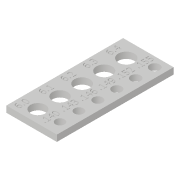
# Autodesk Inventor part: 6mm and number 6 hole test
Saved by Autodesk Inventor 2018 (Build 220112000, 112)
## iProperties
Created: 2019-07-24
Part Number: 6mm and number 6 hole test
Material: Generic
Document SubType Name: Modeling
Designer: ball
Density: 1 g/cm^3
Appearance: Default
Author: ball
Autodesk Inventor part; units mm, degrees
note: some values were not read from the file. Chosen so that the rebuilt part matches the saved one: direction of "Emboss2".
(part 1 of 2)
ref_plane "YZ Plane" through (0, 0, 0) normal (1, 0, 0) x (0, 1, 0)
ref_plane "XZ Plane" through (0, 0, 0) normal (0, 1, 0) x (-1, 0, 0)
ref_plane "XY Plane" through (0, 0, 0) normal (0, 0, 1) x (1, 0, 0)
sketch "Sketch1" plane through (0, 0, 0) normal (0, 1, 0) x (-1, 0, 0)
  line L0 (0, 0) -> (20.32, 0)
  line L1 (20.32, 0) -> (20.32, -46.99)
  line L2 (20.32, -46.99) -> (0, -46.99)
  line L3 (0, -46.99) -> (0, 0)
  circle A0 centre (3.81, -5.08) radius 1.778
  circle A1 centre (3.81, -12.7) radius 1.8161
  circle A2 centre (3.81, -20.32) radius 1.8542
  circle A3 centre (3.81, -27.94) radius 1.8923
  circle A4 centre (3.81, -35.56) radius 1.9304
  circle A5 centre (3.81, -43.18) radius 1.9685
  circle A6 centre (12.7, -5.08) radius 2.9972
  circle A7 centre (12.7, -13.97) radius 3.048
  circle A8 centre (12.7, -22.86) radius 3.0988
  circle A9 centre (12.7, -31.75) radius 3.1496
  circle A10 centre (12.7, -40.64) radius 3.2004
  dimension "d0" = 46.99
  dimension "d1" = 3.556
  dimension "d2" = 5.08
  dimension "d3" = 3.81
  dimension "d4" = 3.6322
  dimension "d5" = 12.7
  dimension "d6" = 3.7084
  dimension "d7" = 3.7846
  dimension "d8" = 3.8608
  dimension "d9" = 3.937
  dimension "d12" = 5.9944
  dimension "d13" = 20.32
  dimension "d14" = 12.7
  dimension "d15" = 5.08
  dimension "d16" = 6.096
  dimension "d17" = 6.1976
  dimension "d18" = 6.2992
  dimension "d19" = 6.4008
  dimension "d20" = 13.97
  dimension "d21" = 22.86
  dimension "d22" = 31.75
  dimension "d23" = 40.64
  dimension "d24" = 43.18
  dimension "d25" = 35.56
  dimension "d26" = 27.94
  dimension "d27" = 20.32
  constraints: 11 centre point, 8 end point, 2 parallel, 1 horizontal, 1 perpendicular
  measures "d0" distance of L0.end L1.end
  measures "d1" diameter of A0
  measures "d2" distance from line of L0 A0.centre
  measures "d3" distance from line of L3 A0.centre
  measures "d4" diameter of A1
  measures "d5" distance from line of L0 A1.centre
  measures "d6" diameter of A2
  measures "d7" diameter of A3
  measures "d8" diameter of A4
  measures "d9" diameter of A5
  measures "d12" diameter of A6
  measures "d13" distance between parallel lines of L3 L1
  measures "d14" distance from line of L3 A6.centre
  measures "d15" distance from line of L0 A6.centre
  measures "d16" diameter of A7
  measures "d17" diameter of A8
  measures "d18" diameter of A9
  measures "d19" diameter of A10
  measures "d20" distance from line of L0 A7.centre
  measures "d21" distance from line of L0 A8.centre
  measures "d22" distance from line of L0 A9.centre
  measures "d23" distance from line of L0 A10.centre
  measures "d24" distance from line of L0 A5.centre
  measures "d25" distance from line of L0 A4.centre
  measures "d26" distance from line of L0 A3.centre
  measures "d27" distance from line of L0 A2.centre
extrude "Extrusion2" add sketch "Sketch1" along normal blind 2.54
sketch "Sketch2" plane through (0, 2.54, 0) normal (0, 1, 0) x (1, 0, 0)
  line L0 (-9.0261, 9.1663) -> (-9.0261, 15.9424) construction
  line L1 (-9.0261, 15.9424) -> (-6.3791, 15.9424) construction
  line L2 (-6.3791, 15.9424) -> (-6.3791, 9.1663) construction
  line L3 (-6.3791, 9.1663) -> (-9.0261, 9.1663) construction
  line L4 (-8.8978, 1.4309) -> (-8.8978, 8.207) construction
  line L5 (-8.8978, 8.207) -> (-6.2508, 8.207) construction
  line L6 (-6.2508, 8.207) -> (-6.2508, 1.4309) construction
  line L7 (-6.2508, 1.4309) -> (-8.8978, 1.4309) construction
  line L8 (-8.9722, 16.6379) -> (-8.9722, 23.414) construction
  line L9 (-8.9722, 23.414) -> (-6.3252, 23.414) construction
  line L10 (-6.3252, 23.414) -> (-6.3252, 16.6379) construction
  line L11 (-6.3252, 16.6379) -> (-8.9722, 16.6379) construction
  line L12 (-9.0872, 24.1029) -> (-9.0872, 30.879) construction
  line L13 (-9.0872, 30.879) -> (-6.4402, 30.879) construction
  line L14 (-6.4402, 30.879) -> (-6.4402, 24.1029) construction
  line L15 (-6.4402, 24.1029) -> (-9.0872, 24.1029) construction
  line L16 (-9.0805, 31.6084) -> (-9.0805, 38.3845) construction
  line L17 (-9.0805, 38.3845) -> (-6.4335, 38.3845) construction
  line L18 (-6.4335, 38.3845) -> (-6.4335, 31.6084) construction
  line L19 (-6.4335, 31.6084) -> (-9.0805, 31.6084) construction
  line L20 (-8.9928, 39.3571) -> (-8.9928, 46.1332) construction
  line L21 (-8.9928, 46.1332) -> (-6.3458, 46.1332) construction
  line L22 (-6.3458, 46.1332) -> (-6.3458, 39.3571) construction
  line L23 (-6.3458, 39.3571) -> (-8.9928, 39.3571) construction
  line L24 (-16.5399, 1.397) -> (-19.1869, 1.397) construction
  line L25 (-19.1869, 1.397) -> (-19.1869, 8.1731) construction
  line L26 (-19.1869, 8.1731) -> (-16.5399, 8.1731) construction
  line L27 (-16.5399, 8.1731) -> (-16.5399, 1.397) construction
  line L28 (-16.5737, 11.213) -> (-19.2208, 11.213) construction
  line L29 (-19.2208, 11.213) -> (-19.2208, 17.9891) construction
  line L30 (-19.2208, 17.9891) -> (-16.5737, 17.9891) construction
  line L31 (-16.5737, 17.9891) -> (-16.5737, 11.213) construction
  line L32 (-16.7292, 20.1372) -> (-19.3762, 20.1372) construction
  line L33 (-19.3762, 20.1372) -> (-19.3762, 26.9133) construction
  line L34 (-19.3762, 26.9133) -> (-16.7292, 26.9133) construction
  line L35 (-16.7292, 26.9133) -> (-16.7292, 20.1372) construction
  line L36 (-16.8036, 29.1425) -> (-19.4506, 29.1425) construction
  line L37 (-19.4506, 29.1425) -> (-19.4506, 35.9186) construction
  line L38 (-19.4506, 35.9186) -> (-16.8036, 35.9186) construction
  line L39 (-16.8036, 35.9186) -> (-16.8036, 29.1425) construction
  line L40 (-16.7564, 38.4315) -> (-19.4034, 38.4315) construction
  line L41 (-19.4034, 38.4315) -> (-19.4034, 45.2076) construction
  line L42 (-19.4034, 45.2076) -> (-16.7564, 45.2076) construction
  line L43 (-16.7564, 45.2076) -> (-16.7564, 38.4315) construction
  spline S0 degree 2 poles (-17.4188, 3.1878) (-17.2232, 3.1878) (-16.8918, 3.0581) (-16.7807, 2.949) knots 0 0 0 1 2 2 2
  spline S1 degree 2 poles (-16.7807, 2.949) (-16.6634, 2.8358) (-16.5419, 2.5518) (-16.5419, 2.3809) knots 0 0 0 1 2 2 2
  spline S2 degree 2 poles (-16.5419, 2.3809) (-16.5419, 2.2101) (-16.6572, 1.9281) (-16.7725, 1.821) knots 0 0 0 1 2 2 2
  spline S3 degree 2 poles (-16.7725, 1.821) (-16.9104, 1.6893) (-17.3735, 1.5411) (-17.7111, 1.5411) knots 0 0 0 1 2 2 2
  spline S4 degree 2 poles (-17.7111, 1.5411) (-18.0425, 1.5411) (-18.5756, 1.677) (-18.7732, 1.819) knots 0 0 0 1 2 2 2
  spline S5 degree 2 poles (-18.7732, 1.819) (-18.9666, 1.9569) (-19.1828, 2.3933) (-19.1828, 2.6794) knots 0 0 0 1 2 2 2
  spline S6 degree 2 poles (-19.1828, 2.6794) (-19.1828, 2.7638) (-19.1663, 2.912) (-19.1478, 2.9675) knots 0 0 0 1 2 2 2
  line L44 (-19.1478, 2.9675) -> (-18.8205, 2.9675)
  line L45 (-18.8205, 2.9675) -> (-18.8205, 2.9531)
  spline S7 degree 2 poles (-18.8205, 2.9531) (-18.8452, 2.9058) (-18.8884, 2.7329) (-18.8884, 2.6341) knots 0 0 0 1 2 2 2
  spline S8 degree 2 poles (-18.8884, 2.6341) (-18.8884, 2.3171) (-18.4603, 1.9281) (-18.0404, 1.891) knots 0 0 0 1 2 2 2
  spline S9 degree 2 poles (-18.0404, 1.891) (-18.1248, 2.0125) (-18.2174, 2.2677) (-18.2174, 2.42) knots 0 0 0 1 2 2 2
  spline S10 degree 2 poles (-18.2174, 2.42) (-18.2174, 2.5682) (-18.1577, 2.7905) (-18.0672, 2.912) knots 0 0 0 1 2 2 2
  spline S11 degree 2 poles (-18.0672, 2.912) (-17.9622, 3.0519) (-17.637, 3.1878) (-17.4188, 3.1878) knots 0 0 0 1 2 2 2
  spline S12 degree 2 poles (-17.4044, 2.842) (-17.5608, 2.842) (-17.7728, 2.7597) (-17.8469, 2.6691) knots 0 0 0 1 2 2 2
  spline S13 degree 2 poles (-17.8469, 2.6691) (-17.9004, 2.6012) (-17.9354, 2.4324) (-17.9354, 2.3439) knots 0 0 0 1 2 2 2
  spline S14 degree 2 poles (-17.9354, 2.3439) (-17.9354, 2.2245) (-17.8634, 2.0001) (-17.7954, 1.891) knots 0 0 0 1 2 2 2
  spline S15 degree 2 poles (-17.7954, 1.891) (-17.7584, 1.889) (-17.6884, 1.8849) (-17.6349, 1.8849) knots 0 0 0 1 2 2 2
  spline S16 degree 2 poles (-17.6349, 1.8849) (-17.3714, 1.8849) (-17.0483, 1.9878) (-16.9639, 2.066) knots 0 0 0 1 2 2 2
  spline S17 degree 2 poles (-16.9639, 2.066) (-16.8836, 2.138) (-16.8198, 2.2945) (-16.8198, 2.383) knots 0 0 0 1 2 2 2
  spline S18 degree 2 poles (-16.8198, 2.383) (-16.8198, 2.5888) (-17.1121, 2.842) (-17.4044, 2.842) knots 0 0 0 1 2 2 2
  line L46 (-16.5954, 4.0338) -> (-16.5954, 3.6262)
  line L47 (-16.5954, 3.6262) -> (-17.0812, 3.6262)
  line L48 (-17.0812, 3.6262) -> (-17.0812, 4.0338)
  line L49 (-17.0812, 4.0338) -> (-16.5954, 4.0338)
  spline S19 degree 2 poles (-17.8654, 6.1271) (-17.1821, 6.1271) (-16.5419, 5.7299) (-16.5419, 5.3161) knots 0 0 0 1 2 2 2
  spline S20 degree 2 poles (-16.5419, 5.3161) (-16.5419, 4.8962) (-17.1944, 4.5031) (-17.8634, 4.5031) knots 0 0 0 1 2 2 2
  spline S21 degree 2 poles (-17.8634, 4.5031) (-18.5509, 4.5031) (-19.1869, 4.9003) (-19.1869, 5.3161) knots 0 0 0 1 2 2 2
  spline S22 degree 2 poles (-19.1869, 5.3161) (-19.1869, 5.734) (-18.5282, 6.1271) (-17.8654, 6.1271) knots 0 0 0 1 2 2 2
  spline S23 degree 2 poles (-17.0915, 5.6907) (-17.2171, 5.7401) (-17.604, 5.7813) (-17.8654, 5.7813) knots 0 0 0 1 2 2 2
  spline S24 degree 2 poles (-17.8654, 5.7813) (-18.1268, 5.7813) (-18.5118, 5.7401) (-18.6414, 5.6887) knots 0 0 0 1 2 2 2
  spline S25 degree 2 poles (-18.6414, 5.6887) (-18.7711, 5.6372) (-18.9049, 5.4581) (-18.9049, 5.3161) knots 0 0 0 1 2 2 2
  spline S26 degree 2 poles (-18.9049, 5.3161) (-18.9049, 5.1741) (-18.7711, 4.9909) (-18.6373, 4.9374) knots 0 0 0 1 2 2 2
  spline S27 degree 2 poles (-18.6373, 4.9374) (-18.5076, 4.8859) (-18.1124, 4.8489) (-17.8634, 4.8489) knots 0 0 0 1 2 2 2
  spline S28 degree 2 poles (-17.8634, 4.8489) (-17.5958, 4.8489) (-17.2376, 4.8818) (-17.0977, 4.9353) knots 0 0 0 1 2 2 2
  spline S29 degree 2 poles (-17.0977, 4.9353) (-16.9659, 4.9847) (-16.8239, 5.1679) (-16.8239, 5.3161) knots 0 0 0 1 2 2 2
  spline S30 degree 2 poles (-16.8239, 5.3161) (-16.8239, 5.4561) (-16.9577, 5.6393) (-17.0915, 5.6907) knots 0 0 0 1 2 2 2
  spline S31 degree 2 poles (-17.4568, 13.0038) (-17.2612, 13.0038) (-16.9298, 12.8741) (-16.8187, 12.765) knots 0 0 0 1 2 2 2
  spline S32 degree 2 poles (-16.8187, 12.765) (-16.7013, 12.6518) (-16.5799, 12.3677) (-16.5799, 12.1969) knots 0 0 0 1 2 2 2
  spline S33 degree 2 poles (-16.5799, 12.1969) (-16.5799, 12.026) (-16.6952, 11.744) (-16.8104, 11.637) knots 0 0 0 1 2 2 2
  spline S34 degree 2 poles (-16.8104, 11.637) (-16.9483, 11.5053) (-17.4115, 11.3571) (-17.749, 11.3571) knots 0 0 0 1 2 2 2
  spline S35 degree 2 poles (-17.749, 11.3571) (-18.0804, 11.3571) (-18.6136, 11.4929) (-18.8112, 11.635) knots 0 0 0 1 2 2 2
  spline S36 degree 2 poles (-18.8112, 11.635) (-19.0046, 11.7729) (-19.2208, 12.2092) (-19.2208, 12.4953) knots 0 0 0 1 2 2 2
  spline S37 degree 2 poles (-19.2208, 12.4953) (-19.2208, 12.5797) (-19.2043, 12.7279) (-19.1858, 12.7835) knots 0 0 0 1 2 2 2
  line L50 (-19.1858, 12.7835) -> (-18.8585, 12.7835)
  line L51 (-18.8585, 12.7835) -> (-18.8585, 12.7691)
  spline S38 degree 2 poles (-18.8585, 12.7691) (-18.8832, 12.7218) (-18.9264, 12.5489) (-18.9264, 12.4501) knots 0 0 0 1 2 2 2
  spline S39 degree 2 poles (-18.9264, 12.4501) (-18.9264, 12.1331) (-18.4983, 11.744) (-18.0784, 11.707) knots 0 0 0 1 2 2 2
  spline S40 degree 2 poles (-18.0784, 11.707) (-18.1628, 11.8284) (-18.2554, 12.0837) (-18.2554, 12.236) knots 0 0 0 1 2 2 2
  spline S41 degree 2 poles (-18.2554, 12.236) (-18.2554, 12.3842) (-18.1957, 12.6065) (-18.1051, 12.7279) knots 0 0 0 1 2 2 2
  spline S42 degree 2 poles (-18.1051, 12.7279) (-18.0002, 12.8679) (-17.6749, 13.0038) (-17.4568, 13.0038) knots 0 0 0 1 2 2 2
  spline S43 degree 2 poles (-17.4424, 12.658) (-17.5988, 12.658) (-17.8108, 12.5756) (-17.8849, 12.4851) knots 0 0 0 1 2 2 2
  spline S44 degree 2 poles (-17.8849, 12.4851) (-17.9384, 12.4171) (-17.9734, 12.2483) (-17.9734, 12.1598) knots 0 0 0 1 2 2 2
  spline S45 degree 2 poles (-17.9734, 12.1598) (-17.9734, 12.0404) (-17.9014, 11.8161) (-17.8334, 11.707) knots 0 0 0 1 2 2 2
  spline S46 degree 2 poles (-17.8334, 11.707) (-17.7964, 11.7049) (-17.7264, 11.7008) (-17.6729, 11.7008) knots 0 0 0 1 2 2 2
  spline S47 degree 2 poles (-17.6729, 11.7008) (-17.4094, 11.7008) (-17.0863, 11.8037) (-17.0019, 11.882) knots 0 0 0 1 2 2 2
  spline S48 degree 2 poles (-17.0019, 11.882) (-16.9216, 11.954) (-16.8578, 12.1104) (-16.8578, 12.1989) knots 0 0 0 1 2 2 2
  spline S49 degree 2 poles (-16.8578, 12.1989) (-16.8578, 12.4048) (-17.1501, 12.658) (-17.4424, 12.658) knots 0 0 0 1 2 2 2
  line L52 (-16.6334, 13.8497) -> (-16.6334, 13.4422)
  line L53 (-16.6334, 13.4422) -> (-17.1192, 13.4422)
  line L54 (-17.1192, 13.4422) -> (-17.1192, 13.8497)
  line L55 (-17.1192, 13.8497) -> (-16.6334, 13.8497)
  line L56 (-16.6334, 15.801) -> (-16.6334, 14.5619)
  line L57 (-16.6334, 14.5619) -> (-16.8928, 14.5619)
  line L58 (-16.8928, 14.5619) -> (-16.8928, 15.023)
  line L59 (-16.8928, 15.023) -> (-18.595, 15.023)
  line L60 (-18.595, 15.023) -> (-18.595, 14.5619)
  line L61 (-18.595, 14.5619) -> (-18.8276, 14.5619)
  spline S50 degree 2 poles (-18.8276, 14.5619) (-18.8276, 14.8233) (-18.9758, 15.0703) (-19.1817, 15.0868) knots 0 0 0 1 2 2 2
  line L62 (-19.1817, 15.0868) -> (-19.1817, 15.3503)
  line L63 (-19.1817, 15.3503) -> (-16.8928, 15.3503)
  line L64 (-16.8928, 15.3503) -> (-16.8928, 15.801)
  line L65 (-16.8928, 15.801) -> (-16.6334, 15.801)
  spline S51 degree 2 poles (-17.6061, 21.928) (-17.4105, 21.928) (-17.0791, 21.7983) (-16.968, 21.6892) knots 0 0 0 1 2 2 2
  spline S52 degree 2 poles (-16.968, 21.6892) (-16.8506, 21.576) (-16.7292, 21.2919) (-16.7292, 21.1211) knots 0 0 0 1 2 2 2
  spline S53 degree 2 poles (-16.7292, 21.1211) (-16.7292, 20.9503) (-16.8445, 20.6683) (-16.9597, 20.5612) knots 0 0 0 1 2 2 2
  spline S54 degree 2 poles (-16.9597, 20.5612) (-17.0976, 20.4295) (-17.5608, 20.2813) (-17.8983, 20.2813) knots 0 0 0 1 2 2 2
  spline S55 degree 2 poles (-17.8983, 20.2813) (-18.2297, 20.2813) (-18.7629, 20.4171) (-18.9605, 20.5592) knots 0 0 0 1 2 2 2
  spline S56 degree 2 poles (-18.9605, 20.5592) (-19.1539, 20.6971) (-19.3701, 21.1334) (-19.3701, 21.4196) knots 0 0 0 1 2 2 2
  spline S57 degree 2 poles (-19.3701, 21.4196) (-19.3701, 21.5039) (-19.3536, 21.6521) (-19.3351, 21.7077) knots 0 0 0 1 2 2 2
  line L66 (-19.3351, 21.7077) -> (-19.0078, 21.7077)
  line L67 (-19.0078, 21.7077) -> (-19.0078, 21.6933)
  spline S58 degree 2 poles (-19.0078, 21.6933) (-19.0325, 21.646) (-19.0757, 21.4731) (-19.0757, 21.3743) knots 0 0 0 1 2 2 2
  spline S59 degree 2 poles (-19.0757, 21.3743) (-19.0757, 21.0573) (-18.6476, 20.6683) (-18.2277, 20.6312) knots 0 0 0 1 2 2 2
  spline S60 degree 2 poles (-18.2277, 20.6312) (-18.3121, 20.7526) (-18.4047, 21.0079) (-18.4047, 21.1602) knots 0 0 0 1 2 2 2
  spline S61 degree 2 poles (-18.4047, 21.1602) (-18.4047, 21.3084) (-18.345, 21.5307) (-18.2544, 21.6521) knots 0 0 0 1 2 2 2
  spline S62 degree 2 poles (-18.2544, 21.6521) (-18.1495, 21.7921) (-17.8242, 21.928) (-17.6061, 21.928) knots 0 0 0 1 2 2 2
  spline S63 degree 2 poles (-17.5917, 21.5822) (-17.7481, 21.5822) (-17.9601, 21.4998) (-18.0342, 21.4093) knots 0 0 0 1 2 2 2
  spline S64 degree 2 poles (-18.0342, 21.4093) (-18.0877, 21.3413) (-18.1227, 21.1726) (-18.1227, 21.084) knots 0 0 0 1 2 2 2
  spline S65 degree 2 poles (-18.1227, 21.084) (-18.1227, 20.9647) (-18.0507, 20.7403) (-17.9827, 20.6312) knots 0 0 0 1 2 2 2
  spline S66 degree 2 poles (-17.9827, 20.6312) (-17.9457, 20.6291) (-17.8757, 20.625) (-17.8222, 20.625) knots 0 0 0 1 2 2 2
  spline S67 degree 2 poles (-17.8222, 20.625) (-17.5587, 20.625) (-17.2356, 20.7279) (-17.1512, 20.8062) knots 0 0 0 1 2 2 2
  spline S68 degree 2 poles (-17.1512, 20.8062) (-17.0709, 20.8782) (-17.0071, 21.0346) (-17.0071, 21.1232) knots 0 0 0 1 2 2 2
  spline S69 degree 2 poles (-17.0071, 21.1232) (-17.0071, 21.329) (-17.2994, 21.5822) (-17.5917, 21.5822) knots 0 0 0 1 2 2 2
  line L68 (-16.7827, 22.7739) -> (-16.7827, 22.3664)
  line L69 (-16.7827, 22.3664) -> (-17.2685, 22.3664)
  line L70 (-17.2685, 22.3664) -> (-17.2685, 22.7739)
  line L71 (-17.2685, 22.7739) -> (-16.7827, 22.7739)
  line L72 (-16.7827, 24.8529) -> (-16.7827, 23.2865)
  line L73 (-16.7827, 23.2865) -> (-17.1429, 23.2865)
  spline S70 degree 2 poles (-17.1429, 23.2865) (-17.3014, 23.4553) (-17.5958, 23.7558) (-17.7543, 23.8999) knots 0 0 0 1 2 2 2
  spline S71 degree 2 poles (-17.7543, 23.8999) (-18.0733, 24.1901) (-18.4562, 24.4021) (-18.6599, 24.4021) knots 0 0 0 1 2 2 2
  spline S72 degree 2 poles (-18.6599, 24.4021) (-18.767, 24.4021) (-18.9275, 24.3362) (-18.979, 24.2765) knots 0 0 0 1 2 2 2
  spline S73 degree 2 poles (-18.979, 24.2765) (-19.0304, 24.2168) (-19.0819, 24.0604) (-19.0819, 23.9657) knots 0 0 0 1 2 2 2
  spline S74 degree 2 poles (-19.0819, 23.9657) (-19.0819, 23.8752) (-19.0366, 23.6899) (-19.0016, 23.6055) knots 0 0 0 1 2 2 2
  spline S75 degree 2 poles (-19.0016, 23.6055) (-18.9728, 23.5335) (-18.8905, 23.3997) (-18.8617, 23.3585) knots 0 0 0 1 2 2 2
  line L74 (-18.8617, 23.3585) -> (-18.8617, 23.34)
  line L75 (-18.8617, 23.34) -> (-19.2239, 23.34)
  spline S76 degree 2 poles (-19.2239, 23.34) (-19.2754, 23.445) (-19.3762, 23.8216) (-19.3762, 23.9904) knots 0 0 0 1 2 2 2
  spline S77 degree 2 poles (-19.3762, 23.9904) (-19.3762, 24.3465) (-18.9996, 24.7479) (-18.6785, 24.7479) knots 0 0 0 1 2 2 2
  spline S78 degree 2 poles (-18.6785, 24.7479) (-18.5282, 24.7479) (-18.2771, 24.6779) (-18.17, 24.6162) knots 0 0 0 1 2 2 2
  spline S79 degree 2 poles (-18.17, 24.6162) (-18.0589, 24.5544) (-17.8407, 24.3753) (-17.7357, 24.2765) knots 0 0 0 1 2 2 2
  spline S80 degree 2 poles (-17.7357, 24.2765) (-17.5608, 24.116) (-17.1862, 23.7228) (-17.0771, 23.6055) knots 0 0 0 1 2 2 2
  line L76 (-17.0771, 23.6055) -> (-17.0771, 24.8529)
  line L77 (-17.0771, 24.8529) -> (-16.7827, 24.8529)
  spline S81 degree 2 poles (-17.6805, 30.9332) (-17.4849, 30.9332) (-17.1535, 30.8036) (-17.0424, 30.6945) knots 0 0 0 1 2 2 2
  spline S82 degree 2 poles (-17.0424, 30.6945) (-16.9251, 30.5813) (-16.8036, 30.2972) (-16.8036, 30.1264) knots 0 0 0 1 2 2 2
  spline S83 degree 2 poles (-16.8036, 30.1264) (-16.8036, 29.9555) (-16.9189, 29.6735) (-17.0341, 29.5665) knots 0 0 0 1 2 2 2
  spline S84 degree 2 poles (-17.0341, 29.5665) (-17.1721, 29.4348) (-17.6352, 29.2866) (-17.9728, 29.2866) knots 0 0 0 1 2 2 2
  spline S85 degree 2 poles (-17.9728, 29.2866) (-18.3041, 29.2866) (-18.8373, 29.4224) (-19.0349, 29.5644) knots 0 0 0 1 2 2 2
  spline S86 degree 2 poles (-19.0349, 29.5644) (-19.2283, 29.7024) (-19.4445, 30.1387) (-19.4445, 30.4248) knots 0 0 0 1 2 2 2
  spline S87 degree 2 poles (-19.4445, 30.4248) (-19.4445, 30.5092) (-19.428, 30.6574) (-19.4095, 30.713) knots 0 0 0 1 2 2 2
  line L78 (-19.4095, 30.713) -> (-19.0822, 30.713)
  line L79 (-19.0822, 30.713) -> (-19.0822, 30.6986)
  spline S88 degree 2 poles (-19.0822, 30.6986) (-19.1069, 30.6512) (-19.1501, 30.4783) (-19.1501, 30.3795) knots 0 0 0 1 2 2 2
  spline S89 degree 2 poles (-19.1501, 30.3795) (-19.1501, 30.0626) (-18.722, 29.6735) (-18.3021, 29.6365) knots 0 0 0 1 2 2 2
  spline S90 degree 2 poles (-18.3021, 29.6365) (-18.3865, 29.7579) (-18.4791, 30.0132) (-18.4791, 30.1655) knots 0 0 0 1 2 2 2
  spline S91 degree 2 poles (-18.4791, 30.1655) (-18.4791, 30.3137) (-18.4194, 30.536) (-18.3288, 30.6574) knots 0 0 0 1 2 2 2
  spline S92 degree 2 poles (-18.3288, 30.6574) (-18.2239, 30.7974) (-17.8987, 30.9332) (-17.6805, 30.9332) knots 0 0 0 1 2 2 2
  spline S93 degree 2 poles (-17.6661, 30.5874) (-17.8225, 30.5874) (-18.0345, 30.5051) (-18.1086, 30.4145) knots 0 0 0 1 2 2 2
  spline S94 degree 2 poles (-18.1086, 30.4145) (-18.1621, 30.3466) (-18.1971, 30.1778) (-18.1971, 30.0893) knots 0 0 0 1 2 2 2
  spline S95 degree 2 poles (-18.1971, 30.0893) (-18.1971, 29.9699) (-18.1251, 29.7456) (-18.0571, 29.6365) knots 0 0 0 1 2 2 2
  spline S96 degree 2 poles (-18.0571, 29.6365) (-18.0201, 29.6344) (-17.9501, 29.6303) (-17.8966, 29.6303) knots 0 0 0 1 2 2 2
  spline S97 degree 2 poles (-17.8966, 29.6303) (-17.6331, 29.6303) (-17.31, 29.7332) (-17.2256, 29.8114) knots 0 0 0 1 2 2 2
  spline S98 degree 2 poles (-17.2256, 29.8114) (-17.1453, 29.8835) (-17.0815, 30.0399) (-17.0815, 30.1284) knots 0 0 0 1 2 2 2
  spline S99 degree 2 poles (-17.0815, 30.1284) (-17.0815, 30.3343) (-17.3738, 30.5874) (-17.6661, 30.5874) knots 0 0 0 1 2 2 2
  line L80 (-16.8571, 31.7792) -> (-16.8571, 31.3717)
  line L81 (-16.8571, 31.3717) -> (-17.3429, 31.3717)
  line L82 (-17.3429, 31.3717) -> (-17.3429, 31.7792)
  line L83 (-17.3429, 31.7792) -> (-16.8571, 31.7792)
  spline S100 degree 2 poles (-19.1563, 32.9772) (-19.1563, 32.8846) (-19.111, 32.7014) (-19.076, 32.6129) knots 0 0 0 1 2 2 2
  spline S101 degree 2 poles (-19.076, 32.6129) (-19.041, 32.5305) (-18.9669, 32.4091) (-18.934, 32.3617) knots 0 0 0 1 2 2 2
  line L84 (-18.934, 32.3617) -> (-18.934, 32.3412)
  line L85 (-18.934, 32.3412) -> (-19.2942, 32.3412)
  spline S102 degree 2 poles (-19.2942, 32.3412) (-19.3539, 32.4523) (-19.4506, 32.8331) (-19.4506, 33.0039) knots 0 0 0 1 2 2 2
  spline S103 degree 2 poles (-19.4506, 33.0039) (-19.4506, 33.1768) (-19.3807, 33.4341) (-19.3066, 33.5391) knots 0 0 0 1 2 2 2
  spline S104 degree 2 poles (-19.3066, 33.5391) (-19.2263, 33.6503) (-18.9937, 33.7655) (-18.8373, 33.7655) knots 0 0 0 1 2 2 2
  spline S105 degree 2 poles (-18.8373, 33.7655) (-18.6273, 33.7655) (-18.3103, 33.4897) (-18.2692, 33.2962) knots 0 0 0 1 2 2 2
  line L86 (-18.2692, 33.2962) -> (-18.2445, 33.2962)
  spline S106 degree 2 poles (-18.2445, 33.2962) (-18.228, 33.3765) (-18.1539, 33.5597) (-18.0798, 33.6379) knots 0 0 0 1 2 2 2
  spline S107 degree 2 poles (-18.0798, 33.6379) (-18.0077, 33.7161) (-17.7772, 33.8149) (-17.6105, 33.8149) knots 0 0 0 1 2 2 2
  spline S108 degree 2 poles (-17.6105, 33.8149) (-17.4396, 33.8149) (-17.1494, 33.6976) (-17.0383, 33.5906) knots 0 0 0 1 2 2 2
  spline S109 degree 2 poles (-17.0383, 33.5906) (-16.923, 33.4794) (-16.8036, 33.1645) (-16.8036, 32.9648) knots 0 0 0 1 2 2 2
  spline S110 degree 2 poles (-16.8036, 32.9648) (-16.8036, 32.7734) (-16.8962, 32.3988) (-16.96, 32.2712) knots 0 0 0 1 2 2 2
  line L87 (-16.96, 32.2712) -> (-17.3203, 32.2712)
  line L88 (-17.3203, 32.2712) -> (-17.3203, 32.2959)
  spline S111 degree 2 poles (-17.3203, 32.2959) (-17.242, 32.4029) (-17.098, 32.7652) (-17.098, 32.9442) knots 0 0 0 1 2 2 2
  spline S112 degree 2 poles (-17.098, 32.9442) (-17.098, 33.0492) (-17.1638, 33.2592) (-17.24, 33.3292) knots 0 0 0 1 2 2 2
  spline S113 degree 2 poles (-17.24, 33.3292) (-17.3161, 33.3971) (-17.4973, 33.4691) (-17.6352, 33.4691) knots 0 0 0 1 2 2 2
  spline S114 degree 2 poles (-17.6352, 33.4691) (-17.7731, 33.4691) (-17.9522, 33.3889) (-18.0036, 33.3168) knots 0 0 0 1 2 2 2
  spline S115 degree 2 poles (-18.0036, 33.3168) (-18.0551, 33.2448) (-18.0942, 33.0492) (-18.0942, 32.934) knots 0 0 0 1 2 2 2
  line L89 (-18.0942, 32.934) -> (-18.0942, 32.7899)
  line L90 (-18.0942, 32.7899) -> (-18.3762, 32.7899)
  line L91 (-18.3762, 32.7899) -> (-18.3762, 32.9031)
  spline S116 degree 2 poles (-18.3762, 32.9031) (-18.3762, 33.1316) (-18.5944, 33.4197) (-18.8023, 33.4197) knots 0 0 0 1 2 2 2
  spline S117 degree 2 poles (-18.8023, 33.4197) (-18.899, 33.4197) (-19.0369, 33.3456) (-19.0781, 33.2859) knots 0 0 0 1 2 2 2
  spline S118 degree 2 poles (-19.0781, 33.2859) (-19.1213, 33.2221) (-19.1563, 33.0657) (-19.1563, 32.9772) knots 0 0 0 1 2 2 2
  spline S119 degree 2 poles (-17.6394, 40.2223) (-17.4439, 40.2223) (-17.1125, 40.0926) (-17.0014, 39.9835) knots 0 0 0 1 2 2 2
  spline S120 degree 2 poles (-17.0014, 39.9835) (-16.884, 39.8703) (-16.7626, 39.5862) (-16.7626, 39.4154) knots 0 0 0 1 2 2 2
  spline S121 degree 2 poles (-16.7626, 39.4154) (-16.7626, 39.2445) (-16.8779, 38.9626) (-16.9931, 38.8555) knots 0 0 0 1 2 2 2
  spline S122 degree 2 poles (-16.9931, 38.8555) (-17.131, 38.7238) (-17.5942, 38.5756) (-17.9317, 38.5756) knots 0 0 0 1 2 2 2
  spline S123 degree 2 poles (-17.9317, 38.5756) (-18.2631, 38.5756) (-18.7962, 38.7114) (-18.9938, 38.8535) knots 0 0 0 1 2 2 2
  spline S124 degree 2 poles (-18.9938, 38.8535) (-19.1873, 38.9914) (-19.4034, 39.4277) (-19.4034, 39.7138) knots 0 0 0 1 2 2 2
  spline S125 degree 2 poles (-19.4034, 39.7138) (-19.4034, 39.7982) (-19.387, 39.9464) (-19.3685, 40.002) knots 0 0 0 1 2 2 2
  line L92 (-19.3685, 40.002) -> (-19.0412, 40.002)
  line L93 (-19.0412, 40.002) -> (-19.0412, 39.9876)
  spline S126 degree 2 poles (-19.0412, 39.9876) (-19.0659, 39.9403) (-19.1091, 39.7674) (-19.1091, 39.6686) knots 0 0 0 1 2 2 2
  spline S127 degree 2 poles (-19.1091, 39.6686) (-19.1091, 39.3516) (-18.681, 38.9626) (-18.2611, 38.9255) knots 0 0 0 1 2 2 2
  spline S128 degree 2 poles (-18.2611, 38.9255) (-18.3455, 39.0469) (-18.4381, 39.3022) (-18.4381, 39.4545) knots 0 0 0 1 2 2 2
  spline S129 degree 2 poles (-18.4381, 39.4545) (-18.4381, 39.6027) (-18.3784, 39.825) (-18.2878, 39.9464) knots 0 0 0 1 2 2 2
  spline S130 degree 2 poles (-18.2878, 39.9464) (-18.1828, 40.0864) (-17.8576, 40.2223) (-17.6394, 40.2223) knots 0 0 0 1 2 2 2
  spline S131 degree 2 poles (-17.625, 39.8765) (-17.7815, 39.8765) (-17.9935, 39.7941) (-18.0676, 39.7036) knots 0 0 0 1 2 2 2
  spline S132 degree 2 poles (-18.0676, 39.7036) (-18.1211, 39.6356) (-18.1561, 39.4668) (-18.1561, 39.3783) knots 0 0 0 1 2 2 2
  spline S133 degree 2 poles (-18.1561, 39.3783) (-18.1561, 39.259) (-18.084, 39.0346) (-18.0161, 38.9255) knots 0 0 0 1 2 2 2
  spline S134 degree 2 poles (-18.0161, 38.9255) (-17.9791, 38.9234) (-17.9091, 38.9193) (-17.8556, 38.9193) knots 0 0 0 1 2 2 2
  spline S135 degree 2 poles (-17.8556, 38.9193) (-17.5921, 38.9193) (-17.2689, 39.0222) (-17.1846, 39.1005) knots 0 0 0 1 2 2 2
  spline S136 degree 2 poles (-17.1846, 39.1005) (-17.1043, 39.1725) (-17.0405, 39.3289) (-17.0405, 39.4174) knots 0 0 0 1 2 2 2
  spline S137 degree 2 poles (-17.0405, 39.4174) (-17.0405, 39.6233) (-17.3328, 39.8765) (-17.625, 39.8765) knots 0 0 0 1 2 2 2
  line L94 (-16.8161, 41.0682) -> (-16.8161, 40.6607)
  line L95 (-16.8161, 40.6607) -> (-17.3019, 40.6607)
  line L96 (-17.3019, 40.6607) -> (-17.3019, 41.0682)
  line L97 (-17.3019, 41.0682) -> (-16.8161, 41.0682)
  line L98 (-17.6888, 43.2151) -> (-17.6888, 42.9125)
  line L99 (-17.6888, 42.9125) -> (-16.8161, 42.9125)
  line L100 (-16.8161, 42.9125) -> (-16.8161, 42.5852)
  line L101 (-16.8161, 42.5852) -> (-17.6888, 42.5852)
  line L102 (-17.6888, 42.5852) -> (-17.6888, 41.4634)
  line L103 (-17.6888, 41.4634) -> (-18.047, 41.4634)
  line L104 (-18.047, 41.4634) -> (-19.3561, 42.5997)
  line L105 (-19.3561, 42.5997) -> (-19.3561, 42.9125)
  line L106 (-19.3561, 42.9125) -> (-17.9626, 42.9125)
  line L107 (-17.9626, 42.9125) -> (-17.9626, 43.2151)
  line L108 (-17.9626, 43.2151) -> (-17.6888, 43.2151)
  line L109 (-17.9626, 42.5852) -> (-18.9547, 42.5852)
  line L110 (-18.9547, 42.5852) -> (-17.9626, 41.731)
  line L111 (-17.9626, 41.731) -> (-17.9626, 42.5852)
  line L112 (-6.4446, 40.0878) -> (-6.4446, 39.6803)
  line L113 (-6.4446, 39.6803) -> (-6.9303, 39.6803)
  line L114 (-6.9303, 39.6803) -> (-6.9303, 40.0878)
  line L115 (-6.9303, 40.0878) -> (-6.4446, 40.0878)
  line L116 (-6.4446, 42.0392) -> (-6.4446, 40.8)
  line L117 (-6.4446, 40.8) -> (-6.7039, 40.8)
  line L118 (-6.7039, 40.8) -> (-6.7039, 41.2611)
  line L119 (-6.7039, 41.2611) -> (-8.4062, 41.2611)
  line L120 (-8.4062, 41.2611) -> (-8.4062, 40.8)
  line L121 (-8.4062, 40.8) -> (-8.6388, 40.8)
  spline S138 degree 2 poles (-8.6388, 40.8) (-8.6388, 41.0614) (-8.787, 41.3084) (-8.9928, 41.3249) knots 0 0 0 1 2 2 2
  line L122 (-8.9928, 41.3249) -> (-8.9928, 41.5884)
  line L123 (-8.9928, 41.5884) -> (-6.7039, 41.5884)
  line L124 (-6.7039, 41.5884) -> (-6.7039, 42.0392)
  line L125 (-6.7039, 42.0392) -> (-6.4446, 42.0392)
  spline S139 degree 2 poles (-7.2514, 44.046) (-7.0682, 44.046) (-6.7554, 43.9287) (-6.6401, 43.8217) knots 0 0 0 1 2 2 2
  spline S140 degree 2 poles (-6.6401, 43.8217) (-6.5248, 43.7146) (-6.391, 43.3956) (-6.391, 43.198) knots 0 0 0 1 2 2 2
  spline S141 degree 2 poles (-6.391, 43.198) (-6.391, 43.0169) (-6.4713, 42.6628) (-6.5351, 42.5332) knots 0 0 0 1 2 2 2
  line L126 (-6.5351, 42.5332) -> (-6.8953, 42.5332)
  line L127 (-6.8953, 42.5332) -> (-6.8953, 42.5579)
  spline S142 degree 2 poles (-6.8953, 42.5579) (-6.8665, 42.597) (-6.7924, 42.7431) (-6.7595, 42.8316) knots 0 0 0 1 2 2 2
  spline S143 degree 2 poles (-6.7595, 42.8316) (-6.7245, 42.9325) (-6.6854, 43.0992) (-6.6854, 43.2042) knots 0 0 0 1 2 2 2
  spline S144 degree 2 poles (-6.6854, 43.2042) (-6.6854, 43.3071) (-6.7595, 43.5006) (-6.8398, 43.5706) knots 0 0 0 1 2 2 2
  spline S145 degree 2 poles (-6.8398, 43.5706) (-6.9159, 43.6344) (-7.1176, 43.7002) (-7.2535, 43.7002) knots 0 0 0 1 2 2 2
  spline S146 degree 2 poles (-7.2535, 43.7002) (-7.3893, 43.7002) (-7.5622, 43.6261) (-7.6199, 43.5562) knots 0 0 0 1 2 2 2
  spline S147 degree 2 poles (-7.6199, 43.5562) (-7.6837, 43.4841) (-7.7372, 43.27) (-7.7372, 43.1404) knots 0 0 0 1 2 2 2
  spline S148 degree 2 poles (-7.7372, 43.1404) (-7.7372, 43.0004) (-7.694, 42.7225) (-7.6755, 42.6381) knots 0 0 0 1 2 2 2
  line L128 (-7.6755, 42.6381) -> (-8.9846, 42.6381)
  line L129 (-8.9846, 42.6381) -> (-8.9846, 44.0316)
  line L130 (-8.9846, 44.0316) -> (-8.6861, 44.0316)
  line L131 (-8.6861, 44.0316) -> (-8.6861, 42.9654)
  line L132 (-8.6861, 42.9654) -> (-8.0089, 42.9654)
  spline S149 degree 2 poles (-8.0089, 42.9654) (-8.0171, 43.0272) (-8.0233, 43.1465) (-8.0233, 43.1959) knots 0 0 0 1 2 2 2
  spline S150 degree 2 poles (-8.0233, 43.1959) (-8.0233, 43.3915) (-7.9595, 43.6611) (-7.8648, 43.7846) knots 0 0 0 1 2 2 2
  spline S151 degree 2 poles (-7.8648, 43.7846) (-7.7701, 43.9102) (-7.482, 44.046) (-7.2514, 44.046) knots 0 0 0 1 2 2 2
  spline S152 degree 2 poles (-7.2514, 45.9521) (-7.0682, 45.9521) (-6.7554, 45.8347) (-6.6401, 45.7277) knots 0 0 0 1 2 2 2
  spline S153 degree 2 poles (-6.6401, 45.7277) (-6.5248, 45.6207) (-6.391, 45.3016) (-6.391, 45.104) knots 0 0 0 1 2 2 2
  spline S154 degree 2 poles (-6.391, 45.104) (-6.391, 44.9229) (-6.4713, 44.5689) (-6.5351, 44.4392) knots 0 0 0 1 2 2 2
  line L133 (-6.5351, 44.4392) -> (-6.8953, 44.4392)
  line L134 (-6.8953, 44.4392) -> (-6.8953, 44.4639)
  spline S155 degree 2 poles (-6.8953, 44.4639) (-6.8665, 44.503) (-6.7924, 44.6491) (-6.7595, 44.7376) knots 0 0 0 1 2 2 2
  spline S156 degree 2 poles (-6.7595, 44.7376) (-6.7245, 44.8385) (-6.6854, 45.0052) (-6.6854, 45.1102) knots 0 0 0 1 2 2 2
  spline S157 degree 2 poles (-6.6854, 45.1102) (-6.6854, 45.2131) (-6.7595, 45.4066) (-6.8398, 45.4766) knots 0 0 0 1 2 2 2
  spline S158 degree 2 poles (-6.8398, 45.4766) (-6.9159, 45.5404) (-7.1176, 45.6063) (-7.2535, 45.6063) knots 0 0 0 1 2 2 2
  spline S159 degree 2 poles (-7.2535, 45.6063) (-7.3893, 45.6063) (-7.5622, 45.5322) (-7.6199, 45.4622) knots 0 0 0 1 2 2 2
  spline S160 degree 2 poles (-7.6199, 45.4622) (-7.6837, 45.3901) (-7.7372, 45.1761) (-7.7372, 45.0464) knots 0 0 0 1 2 2 2
  spline S161 degree 2 poles (-7.7372, 45.0464) (-7.7372, 44.9064) (-7.694, 44.6286) (-7.6755, 44.5442) knots 0 0 0 1 2 2 2
  line L135 (-7.6755, 44.5442) -> (-8.9846, 44.5442)
  line L136 (-8.9846, 44.5442) -> (-8.9846, 45.9377)
  line L137 (-8.9846, 45.9377) -> (-8.6861, 45.9377)
  line L138 (-8.6861, 45.9377) -> (-8.6861, 44.8714)
  line L139 (-8.6861, 44.8714) -> (-8.0089, 44.8714)
  spline S162 degree 2 poles (-8.0089, 44.8714) (-8.0171, 44.9332) (-8.0233, 45.0526) (-8.0233, 45.102) knots 0 0 0 1 2 2 2
  spline S163 degree 2 poles (-8.0233, 45.102) (-8.0233, 45.2975) (-7.9595, 45.5672) (-7.8648, 45.6907) knots 0 0 0 1 2 2 2
  spline S164 degree 2 poles (-7.8648, 45.6907) (-7.7701, 45.8162) (-7.482, 45.9521) (-7.2514, 45.9521) knots 0 0 0 1 2 2 2
  line L140 (-6.487, 32.3391) -> (-6.487, 31.9316)
  line L141 (-6.487, 31.9316) -> (-6.9728, 31.9316)
  line L142 (-6.9728, 31.9316) -> (-6.9728, 32.3391)
  line L143 (-6.9728, 32.3391) -> (-6.487, 32.3391)
  line L144 (-6.487, 34.2904) -> (-6.487, 33.0513)
  line L145 (-6.487, 33.0513) -> (-6.7464, 33.0513)
  line L146 (-6.7464, 33.0513) -> (-6.7464, 33.5124)
  line L147 (-6.7464, 33.5124) -> (-8.4486, 33.5124)
  line L148 (-8.4486, 33.5124) -> (-8.4486, 33.0513)
  line L149 (-8.4486, 33.0513) -> (-8.6812, 33.0513)
  spline S165 degree 2 poles (-8.6812, 33.0513) (-8.6812, 33.3127) (-8.8294, 33.5597) (-9.0352, 33.5762) knots 0 0 0 1 2 2 2
  line L150 (-9.0352, 33.5762) -> (-9.0352, 33.8397)
  line L151 (-9.0352, 33.8397) -> (-6.7464, 33.8397)
  line L152 (-6.7464, 33.8397) -> (-6.7464, 34.2904)
  line L153 (-6.7464, 34.2904) -> (-6.487, 34.2904)
  spline S166 degree 2 poles (-7.2939, 36.2973) (-7.1107, 36.2973) (-6.7978, 36.18) (-6.6826, 36.073) knots 0 0 0 1 2 2 2
  spline S167 degree 2 poles (-6.6826, 36.073) (-6.5673, 35.9659) (-6.4335, 35.6469) (-6.4335, 35.4493) knots 0 0 0 1 2 2 2
  spline S168 degree 2 poles (-6.4335, 35.4493) (-6.4335, 35.2682) (-6.5138, 34.9141) (-6.5776, 34.7844) knots 0 0 0 1 2 2 2
  line L154 (-6.5776, 34.7844) -> (-6.9378, 34.7844)
  line L155 (-6.9378, 34.7844) -> (-6.9378, 34.8091)
  spline S169 degree 2 poles (-6.9378, 34.8091) (-6.909, 34.8482) (-6.8349, 34.9944) (-6.8019, 35.0829) knots 0 0 0 1 2 2 2
  spline S170 degree 2 poles (-6.8019, 35.0829) (-6.7669, 35.1838) (-6.7278, 35.3505) (-6.7278, 35.4555) knots 0 0 0 1 2 2 2
  spline S171 degree 2 poles (-6.7278, 35.4555) (-6.7278, 35.5584) (-6.8019, 35.7519) (-6.8822, 35.8218) knots 0 0 0 1 2 2 2
  spline S172 degree 2 poles (-6.8822, 35.8218) (-6.9584, 35.8857) (-7.1601, 35.9515) (-7.2959, 35.9515) knots 0 0 0 1 2 2 2
  spline S173 degree 2 poles (-7.2959, 35.9515) (-7.4318, 35.9515) (-7.6047, 35.8774) (-7.6623, 35.8074) knots 0 0 0 1 2 2 2
  spline S174 degree 2 poles (-7.6623, 35.8074) (-7.7261, 35.7354) (-7.7797, 35.5213) (-7.7797, 35.3917) knots 0 0 0 1 2 2 2
  spline S175 degree 2 poles (-7.7797, 35.3917) (-7.7797, 35.2517) (-7.7364, 34.9738) (-7.7179, 34.8894) knots 0 0 0 1 2 2 2
  line L156 (-7.7179, 34.8894) -> (-9.027, 34.8894)
  line L157 (-9.027, 34.8894) -> (-9.027, 36.2829)
  line L158 (-9.027, 36.2829) -> (-8.7285, 36.2829)
  line L159 (-8.7285, 36.2829) -> (-8.7285, 35.2167)
  line L160 (-8.7285, 35.2167) -> (-8.0514, 35.2167)
  spline S176 degree 2 poles (-8.0514, 35.2167) (-8.0596, 35.2784) (-8.0658, 35.3978) (-8.0658, 35.4472) knots 0 0 0 1 2 2 2
  spline S177 degree 2 poles (-8.0658, 35.4472) (-8.0658, 35.6428) (-8.002, 35.9124) (-7.9073, 36.0359) knots 0 0 0 1 2 2 2
  spline S178 degree 2 poles (-7.9073, 36.0359) (-7.8126, 36.1615) (-7.5244, 36.2973) (-7.2939, 36.2973) knots 0 0 0 1 2 2 2
  line L161 (-6.487, 38.2301) -> (-6.487, 36.6637)
  line L162 (-6.487, 36.6637) -> (-6.8472, 36.6637)
  spline S179 degree 2 poles (-6.8472, 36.6637) (-7.0057, 36.8325) (-7.3001, 37.133) (-7.4585, 37.2771) knots 0 0 0 1 2 2 2
  spline S180 degree 2 poles (-7.4585, 37.2771) (-7.7776, 37.5673) (-8.1604, 37.7793) (-8.3642, 37.7793) knots 0 0 0 1 2 2 2
  spline S181 degree 2 poles (-8.3642, 37.7793) (-8.4713, 37.7793) (-8.6318, 37.7135) (-8.6833, 37.6538) knots 0 0 0 1 2 2 2
  spline S182 degree 2 poles (-8.6833, 37.6538) (-8.7347, 37.5941) (-8.7862, 37.4376) (-8.7862, 37.343) knots 0 0 0 1 2 2 2
  spline S183 degree 2 poles (-8.7862, 37.343) (-8.7862, 37.2524) (-8.7409, 37.0671) (-8.7059, 36.9828) knots 0 0 0 1 2 2 2
  spline S184 degree 2 poles (-8.7059, 36.9828) (-8.6771, 36.9107) (-8.5948, 36.7769) (-8.5659, 36.7358) knots 0 0 0 1 2 2 2
  line L163 (-8.5659, 36.7358) -> (-8.5659, 36.7172)
  line L164 (-8.5659, 36.7172) -> (-8.9282, 36.7172)
  spline S185 degree 2 poles (-8.9282, 36.7172) (-8.9797, 36.8222) (-9.0805, 37.1989) (-9.0805, 37.3677) knots 0 0 0 1 2 2 2
  spline S186 degree 2 poles (-9.0805, 37.3677) (-9.0805, 37.7238) (-8.7038, 38.1251) (-8.3827, 38.1251) knots 0 0 0 1 2 2 2
  spline S187 degree 2 poles (-8.3827, 38.1251) (-8.2325, 38.1251) (-7.9814, 38.0552) (-7.8743, 37.9934) knots 0 0 0 1 2 2 2
  spline S188 degree 2 poles (-7.8743, 37.9934) (-7.7632, 37.9317) (-7.545, 37.7526) (-7.44, 37.6538) knots 0 0 0 1 2 2 2
  spline S189 degree 2 poles (-7.44, 37.6538) (-7.2651, 37.4932) (-6.8904, 37.1001) (-6.7814, 36.9828) knots 0 0 0 1 2 2 2
  line L165 (-6.7814, 36.9828) -> (-6.7814, 38.2301)
  line L166 (-6.7814, 38.2301) -> (-6.487, 38.2301)
  line L167 (-6.4957, 24.8336) -> (-6.4957, 24.4261)
  line L168 (-6.4957, 24.4261) -> (-6.9815, 24.4261)
  line L169 (-6.9815, 24.4261) -> (-6.9815, 24.8336)
  line L170 (-6.9815, 24.8336) -> (-6.4957, 24.8336)
  line L171 (-6.4957, 26.7849) -> (-6.4957, 25.5458)
  line L172 (-6.4957, 25.5458) -> (-6.7551, 25.5458)
  line L173 (-6.7551, 25.5458) -> (-6.7551, 26.0069)
  line L174 (-6.7551, 26.0069) -> (-8.4573, 26.0069)
  line L175 (-8.4573, 26.0069) -> (-8.4573, 25.5458)
  line L176 (-8.4573, 25.5458) -> (-8.6899, 25.5458)
  spline S190 degree 2 poles (-8.6899, 25.5458) (-8.6899, 25.8072) (-8.8381, 26.0542) (-9.044, 26.0707) knots 0 0 0 1 2 2 2
  line L177 (-9.044, 26.0707) -> (-9.044, 26.3342)
  line L178 (-9.044, 26.3342) -> (-6.7551, 26.3342)
  line L179 (-6.7551, 26.3342) -> (-6.7551, 26.7849)
  line L180 (-6.7551, 26.7849) -> (-6.4957, 26.7849)
  line L181 (-7.3685, 28.8865) -> (-7.3685, 28.5839)
  line L182 (-7.3685, 28.5839) -> (-6.4957, 28.5839)
  line L183 (-6.4957, 28.5839) -> (-6.4957, 28.2566)
  line L184 (-6.4957, 28.2566) -> (-7.3685, 28.2566)
  line L185 (-7.3685, 28.2566) -> (-7.3685, 27.1348)
  line L186 (-7.3685, 27.1348) -> (-7.7266, 27.1348)
  line L187 (-7.7266, 27.1348) -> (-9.0357, 28.2711)
  line L188 (-9.0357, 28.2711) -> (-9.0357, 28.5839)
  line L189 (-9.0357, 28.5839) -> (-7.6422, 28.5839)
  line L190 (-7.6422, 28.5839) -> (-7.6422, 28.8865)
  line L191 (-7.6422, 28.8865) -> (-7.3685, 28.8865)
  line L192 (-7.6422, 28.2566) -> (-8.6344, 28.2566)
  line L193 (-8.6344, 28.2566) -> (-7.6422, 27.4024)
  line L194 (-7.6422, 27.4024) -> (-7.6422, 28.2566)
  spline S191 degree 2 poles (-8.2103, 29.0882) (-8.4059, 29.0882) (-8.7311, 29.2158) (-8.8484, 29.327) knots 0 0 0 1 2 2 2
  spline S192 degree 2 poles (-8.8484, 29.327) (-8.9616, 29.432) (-9.0872, 29.7387) (-9.0872, 29.8951) knots 0 0 0 1 2 2 2
  spline S193 degree 2 poles (-9.0872, 29.8951) (-9.0872, 30.0701) (-8.9699, 30.3541) (-8.8587, 30.4591) knots 0 0 0 1 2 2 2
  spline S194 degree 2 poles (-8.8587, 30.4591) (-8.7187, 30.5908) (-8.2659, 30.7349) (-7.918, 30.7349) knots 0 0 0 1 2 2 2
  spline S195 degree 2 poles (-7.918, 30.7349) (-7.6031, 30.7349) (-7.0391, 30.5929) (-6.8518, 30.455) knots 0 0 0 1 2 2 2
  spline S196 degree 2 poles (-6.8518, 30.455) (-6.6542, 30.3088) (-6.4463, 29.8971) (-6.4463, 29.5966) knots 0 0 0 1 2 2 2
  spline S197 degree 2 poles (-6.4463, 29.5966) (-6.4463, 29.5287) (-6.4607, 29.3743) (-6.4813, 29.3085) knots 0 0 0 1 2 2 2
  line L195 (-6.4813, 29.3085) -> (-6.8086, 29.3085)
  line L196 (-6.8086, 29.3085) -> (-6.8086, 29.3249)
  spline S198 degree 2 poles (-6.8086, 29.3249) (-6.7839, 29.3682) (-6.7407, 29.5493) (-6.7407, 29.6419) knots 0 0 0 1 2 2 2
  spline S199 degree 2 poles (-6.7407, 29.6419) (-6.7407, 29.9754) (-7.1812, 30.3562) (-7.5887, 30.3829) knots 0 0 0 1 2 2 2
  spline S200 degree 2 poles (-7.5887, 30.3829) (-7.4961, 30.2471) (-7.4117, 30.0001) (-7.4117, 29.8539) knots 0 0 0 1 2 2 2
  spline S201 degree 2 poles (-7.4117, 29.8539) (-7.4117, 29.714) (-7.4734, 29.4814) (-7.562, 29.364) knots 0 0 0 1 2 2 2
  spline S202 degree 2 poles (-7.562, 29.364) (-7.6669, 29.2282) (-7.986, 29.0882) (-8.2103, 29.0882) knots 0 0 0 1 2 2 2
  spline S203 degree 2 poles (-7.9942, 30.3912) (-8.2515, 30.3912) (-8.5767, 30.2965) (-8.6652, 30.2121) knots 0 0 0 1 2 2 2
  spline S204 degree 2 poles (-8.6652, 30.2121) (-8.7476, 30.138) (-8.8093, 29.9836) (-8.8093, 29.893) knots 0 0 0 1 2 2 2
  spline S205 degree 2 poles (-8.8093, 29.893) (-8.8093, 29.6831) (-8.5088, 29.434) (-8.2247, 29.434) knots 0 0 0 1 2 2 2
  spline S206 degree 2 poles (-8.2247, 29.434) (-8.0642, 29.434) (-7.8563, 29.5164) (-7.7822, 29.6069) knots 0 0 0 1 2 2 2
  spline S207 degree 2 poles (-7.7822, 29.6069) (-7.7287, 29.6728) (-7.6937, 29.8354) (-7.6937, 29.9301) knots 0 0 0 1 2 2 2
  spline S208 degree 2 poles (-7.6937, 29.9301) (-7.6937, 30.0392) (-7.7698, 30.2903) (-7.8337, 30.385) knots 0 0 0 1 2 2 2
  spline S209 degree 2 poles (-7.8337, 30.385) (-7.8584, 30.387) (-7.9427, 30.3912) (-7.9942, 30.3912) knots 0 0 0 1 2 2 2
  line L197 (-6.3849, 17.3686) -> (-6.3849, 16.9611)
  line L198 (-6.3849, 16.9611) -> (-6.8707, 16.9611)
  line L199 (-6.8707, 16.9611) -> (-6.8707, 17.3686)
  line L200 (-6.8707, 17.3686) -> (-6.3849, 17.3686)
  line L201 (-6.3849, 19.32) -> (-6.3849, 18.0808)
  line L202 (-6.3849, 18.0808) -> (-6.6443, 18.0808)
  line L203 (-6.6443, 18.0808) -> (-6.6443, 18.5419)
  line L204 (-6.6443, 18.5419) -> (-8.3465, 18.5419)
  line L205 (-8.3465, 18.5419) -> (-8.3465, 18.0808)
  line L206 (-8.3465, 18.0808) -> (-8.5791, 18.0808)
  spline S210 degree 2 poles (-8.5791, 18.0808) (-8.5791, 18.3422) (-8.7273, 18.5892) (-8.9331, 18.6057) knots 0 0 0 1 2 2 2
  line L207 (-8.9331, 18.6057) -> (-8.9331, 18.8692)
  line L208 (-8.9331, 18.8692) -> (-6.6443, 18.8692)
  line L209 (-6.6443, 18.8692) -> (-6.6443, 19.32)
  line L210 (-6.6443, 19.32) -> (-6.3849, 19.32)
  line L211 (-7.2576, 21.4215) -> (-7.2576, 21.1189)
  line L212 (-7.2576, 21.1189) -> (-6.3849, 21.1189)
  line L213 (-6.3849, 21.1189) -> (-6.3849, 20.7917)
  line L214 (-6.3849, 20.7917) -> (-7.2576, 20.7917)
  line L215 (-7.2576, 20.7917) -> (-7.2576, 19.6699)
  line L216 (-7.2576, 19.6699) -> (-7.6158, 19.6699)
  line L217 (-7.6158, 19.6699) -> (-8.9249, 20.8061)
  line L218 (-8.9249, 20.8061) -> (-8.9249, 21.1189)
  line L219 (-8.9249, 21.1189) -> (-7.5314, 21.1189)
  line L220 (-7.5314, 21.1189) -> (-7.5314, 21.4215)
  line L221 (-7.5314, 21.4215) -> (-7.2576, 21.4215)
  line L222 (-7.5314, 20.7917) -> (-8.5235, 20.7917)
  line L223 (-8.5235, 20.7917) -> (-7.5314, 19.9375)
  line L224 (-7.5314, 19.9375) -> (-7.5314, 20.7917)
  spline S211 degree 2 poles (-7.2082, 23.2987) (-7.0127, 23.2987) (-6.6813, 23.1691) (-6.5702, 23.06) knots 0 0 0 1 2 2 2
  spline S212 degree 2 poles (-6.5702, 23.06) (-6.4528, 22.9468) (-6.3314, 22.6627) (-6.3314, 22.4919) knots 0 0 0 1 2 2 2
  spline S213 degree 2 poles (-6.3314, 22.4919) (-6.3314, 22.321) (-6.4467, 22.039) (-6.5619, 21.932) knots 0 0 0 1 2 2 2
  spline S214 degree 2 poles (-6.5619, 21.932) (-6.6998, 21.8003) (-7.163, 21.6521) (-7.5005, 21.6521) knots 0 0 0 1 2 2 2
  spline S215 degree 2 poles (-7.5005, 21.6521) (-7.8319, 21.6521) (-8.365, 21.7879) (-8.5626, 21.9299) knots 0 0 0 1 2 2 2
  spline S216 degree 2 poles (-8.5626, 21.9299) (-8.7561, 22.0678) (-8.9722, 22.5042) (-8.9722, 22.7903) knots 0 0 0 1 2 2 2
  spline S217 degree 2 poles (-8.9722, 22.7903) (-8.9722, 22.8747) (-8.9558, 23.0229) (-8.9373, 23.0785) knots 0 0 0 1 2 2 2
  line L225 (-8.9373, 23.0785) -> (-8.61, 23.0785)
  line L226 (-8.61, 23.0785) -> (-8.61, 23.0641)
  spline S218 degree 2 poles (-8.61, 23.0641) (-8.6347, 23.0167) (-8.6779, 22.8438) (-8.6779, 22.745) knots 0 0 0 1 2 2 2
  spline S219 degree 2 poles (-8.6779, 22.745) (-8.6779, 22.4281) (-8.2498, 22.039) (-7.8299, 22.002) knots 0 0 0 1 2 2 2
  spline S220 degree 2 poles (-7.8299, 22.002) (-7.9143, 22.1234) (-8.0069, 22.3787) (-8.0069, 22.531) knots 0 0 0 1 2 2 2
  spline S221 degree 2 poles (-8.0069, 22.531) (-8.0069, 22.6792) (-7.9472, 22.9015) (-7.8566, 23.0229) knots 0 0 0 1 2 2 2
  spline S222 degree 2 poles (-7.8566, 23.0229) (-7.7516, 23.1629) (-7.4264, 23.2987) (-7.2082, 23.2987) knots 0 0 0 1 2 2 2
  spline S223 degree 2 poles (-7.1938, 22.9529) (-7.3503, 22.9529) (-7.5623, 22.8706) (-7.6364, 22.78) knots 0 0 0 1 2 2 2
  spline S224 degree 2 poles (-7.6364, 22.78) (-7.6899, 22.7121) (-7.7249, 22.5433) (-7.7249, 22.4548) knots 0 0 0 1 2 2 2
  spline S225 degree 2 poles (-7.7249, 22.4548) (-7.7249, 22.3354) (-7.6528, 22.1111) (-7.5849, 22.002) knots 0 0 0 1 2 2 2
  spline S226 degree 2 poles (-7.5849, 22.002) (-7.5479, 21.9999) (-7.4779, 21.9958) (-7.4244, 21.9958) knots 0 0 0 1 2 2 2
  spline S227 degree 2 poles (-7.4244, 21.9958) (-7.1609, 21.9958) (-6.8377, 22.0987) (-6.7533, 22.1769) knots 0 0 0 1 2 2 2
  spline S228 degree 2 poles (-6.7533, 22.1769) (-6.6731, 22.249) (-6.6093, 22.4054) (-6.6093, 22.4939) knots 0 0 0 1 2 2 2
  spline S229 degree 2 poles (-6.6093, 22.4939) (-6.6093, 22.6998) (-6.9016, 22.9529) (-7.1938, 22.9529) knots 0 0 0 1 2 2 2
  line L227 (-6.4326, 9.897) -> (-6.4326, 9.4895)
  line L228 (-6.4326, 9.4895) -> (-6.9184, 9.4895)
  line L229 (-6.9184, 9.4895) -> (-6.9184, 9.897)
  line L230 (-6.9184, 9.897) -> (-6.4326, 9.897)
  line L231 (-6.4326, 11.8483) -> (-6.4326, 10.6092)
  line L232 (-6.4326, 10.6092) -> (-6.6919, 10.6092)
  line L233 (-6.6919, 10.6092) -> (-6.6919, 11.0703)
  line L234 (-6.6919, 11.0703) -> (-8.3942, 11.0703)
  line L235 (-8.3942, 11.0703) -> (-8.3942, 10.6092)
  line L236 (-8.3942, 10.6092) -> (-8.6268, 10.6092)
  spline S230 degree 2 poles (-8.6268, 10.6092) (-8.6268, 10.8706) (-8.775, 11.1176) (-8.9808, 11.1341) knots 0 0 0 1 2 2 2
  line L237 (-8.9808, 11.1341) -> (-8.9808, 11.3975)
  line L238 (-8.9808, 11.3975) -> (-6.6919, 11.3975)
  line L239 (-6.6919, 11.3975) -> (-6.6919, 11.8483)
  line L240 (-6.6919, 11.8483) -> (-6.4326, 11.8483)
  line L241 (-7.3053, 13.9499) -> (-7.3053, 13.6473)
  line L242 (-7.3053, 13.6473) -> (-6.4326, 13.6473)
  line L243 (-6.4326, 13.6473) -> (-6.4326, 13.32)
  line L244 (-6.4326, 13.32) -> (-7.3053, 13.32)
  line L245 (-7.3053, 13.32) -> (-7.3053, 12.1982)
  line L246 (-7.3053, 12.1982) -> (-7.6635, 12.1982)
  line L247 (-7.6635, 12.1982) -> (-8.9726, 13.3344)
  line L248 (-8.9726, 13.3344) -> (-8.9726, 13.6473)
  line L249 (-8.9726, 13.6473) -> (-7.5791, 13.6473)
  line L250 (-7.5791, 13.6473) -> (-7.5791, 13.9499)
  line L251 (-7.5791, 13.9499) -> (-7.3053, 13.9499)
  line L252 (-7.5791, 13.32) -> (-8.5712, 13.32)
  line L253 (-8.5712, 13.32) -> (-7.5791, 12.4658)
  line L254 (-7.5791, 12.4658) -> (-7.5791, 13.32)
  spline S231 degree 2 poles (-8.7318, 14.907) (-8.7318, 14.8144) (-8.6865, 14.6312) (-8.6515, 14.5427) knots 0 0 0 1 2 2 2
  spline S232 degree 2 poles (-8.6515, 14.5427) (-8.6165, 14.4604) (-8.5424, 14.3389) (-8.5095, 14.2916) knots 0 0 0 1 2 2 2
  line L255 (-8.5095, 14.2916) -> (-8.5095, 14.271)
  line L256 (-8.5095, 14.271) -> (-8.8697, 14.271)
  spline S233 degree 2 poles (-8.8697, 14.271) (-8.9294, 14.3821) (-9.0261, 14.7629) (-9.0261, 14.9338) knots 0 0 0 1 2 2 2
  spline S234 degree 2 poles (-9.0261, 14.9338) (-9.0261, 15.1067) (-8.9561, 15.364) (-8.882, 15.469) knots 0 0 0 1 2 2 2
  spline S235 degree 2 poles (-8.882, 15.469) (-8.8017, 15.5801) (-8.5692, 15.6954) (-8.4127, 15.6954) knots 0 0 0 1 2 2 2
  spline S236 degree 2 poles (-8.4127, 15.6954) (-8.2028, 15.6954) (-7.8858, 15.4196) (-7.8446, 15.2261) knots 0 0 0 1 2 2 2
  line L257 (-7.8446, 15.2261) -> (-7.8199, 15.2261)
  spline S237 degree 2 poles (-7.8199, 15.2261) (-7.8034, 15.3063) (-7.7293, 15.4895) (-7.6552, 15.5678) knots 0 0 0 1 2 2 2
  spline S238 degree 2 poles (-7.6552, 15.5678) (-7.5832, 15.646) (-7.3527, 15.7448) (-7.1859, 15.7448) knots 0 0 0 1 2 2 2
  spline S239 degree 2 poles (-7.1859, 15.7448) (-7.0151, 15.7448) (-6.7249, 15.6274) (-6.6137, 15.5204) knots 0 0 0 1 2 2 2
  spline S240 degree 2 poles (-6.6137, 15.5204) (-6.4985, 15.4093) (-6.3791, 15.0943) (-6.3791, 14.8947) knots 0 0 0 1 2 2 2
  spline S241 degree 2 poles (-6.3791, 14.8947) (-6.3791, 14.7032) (-6.4717, 14.3286) (-6.5355, 14.201) knots 0 0 0 1 2 2 2
  line L258 (-6.5355, 14.201) -> (-6.8957, 14.201)
  line L259 (-6.8957, 14.201) -> (-6.8957, 14.2257)
  spline S242 degree 2 poles (-6.8957, 14.2257) (-6.8175, 14.3327) (-6.6734, 14.695) (-6.6734, 14.8741) knots 0 0 0 1 2 2 2
  spline S243 degree 2 poles (-6.6734, 14.8741) (-6.6734, 14.9791) (-6.7393, 15.189) (-6.8154, 15.259) knots 0 0 0 1 2 2 2
  spline S244 degree 2 poles (-6.8154, 15.259) (-6.8916, 15.3269) (-7.0727, 15.399) (-7.2106, 15.399) knots 0 0 0 1 2 2 2
  spline S245 degree 2 poles (-7.2106, 15.399) (-7.3486, 15.399) (-7.5276, 15.3187) (-7.5791, 15.2466) knots 0 0 0 1 2 2 2
  spline S246 degree 2 poles (-7.5791, 15.2466) (-7.6305, 15.1746) (-7.6697, 14.9791) (-7.6697, 14.8638) knots 0 0 0 1 2 2 2
  line L260 (-7.6697, 14.8638) -> (-7.6697, 14.7197)
  line L261 (-7.6697, 14.7197) -> (-7.9516, 14.7197)
  line L262 (-7.9516, 14.7197) -> (-7.9516, 14.8329)
  spline S247 degree 2 poles (-7.9516, 14.8329) (-7.9516, 15.0614) (-8.1698, 15.3496) (-8.3777, 15.3496) knots 0 0 0 1 2 2 2
  spline S248 degree 2 poles (-8.3777, 15.3496) (-8.4745, 15.3496) (-8.6124, 15.2755) (-8.6535, 15.2158) knots 0 0 0 1 2 2 2
  spline S249 degree 2 poles (-8.6535, 15.2158) (-8.6968, 15.152) (-8.7318, 14.9955) (-8.7318, 14.907) knots 0 0 0 1 2 2 2
  line L263 (-6.3064, 2.1616) -> (-6.3064, 1.7541)
  line L264 (-6.3064, 1.7541) -> (-6.7922, 1.7541)
  line L265 (-6.7922, 1.7541) -> (-6.7922, 2.1616)
  line L266 (-6.7922, 2.1616) -> (-6.3064, 2.1616)
  line L267 (-6.3064, 4.1129) -> (-6.3064, 2.8738)
  line L268 (-6.3064, 2.8738) -> (-6.5657, 2.8738)
  line L269 (-6.5657, 2.8738) -> (-6.5657, 3.3349)
  line L270 (-6.5657, 3.3349) -> (-8.268, 3.3349)
  line L271 (-8.268, 3.3349) -> (-8.268, 2.8738)
  line L272 (-8.268, 2.8738) -> (-8.5006, 2.8738)
  spline S250 degree 2 poles (-8.5006, 2.8738) (-8.5006, 3.1352) (-8.6488, 3.3822) (-8.8546, 3.3987) knots 0 0 0 1 2 2 2